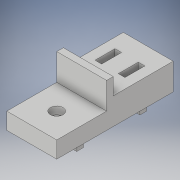
# Autodesk Inventor part: FixedFiber
Saved by Autodesk Inventor 2019 (Build 230136000, 136)
## iProperties
Created: 2019-06-10
Part Number: FixedFiber
Material: Generic
Document SubType Name: Modeling
Designer: aorfi
Density: 1 g/cm^3
Appearance: Default
Author: aorfi
Autodesk Inventor part; units mm, degrees
ref_plane "YZ Plane" through (0, 0, 0) normal (1, 0, 0) x (0, 1, 0)
ref_plane "XZ Plane" through (0, 0, 0) normal (0, 1, 0) x (-1, 0, 0)
ref_plane "XY Plane" through (0, 0, 0) normal (0, 0, 1) x (1, 0, 0)
sketch "Sketch1" plane through (0, 0, 0) normal (0, 1, 0) x (-1, 0, 0)
  line L0 (-7.5, 17.5) -> (7.5, 17.5)
  line L1 (7.5, 17.5) -> (7.5, -17.5)
  line L2 (7.5, -17.5) -> (-7.5, -17.5)
  line L3 (-7.5, -17.5) -> (-7.5, 17.5)
  line L4 (-7.5, 17.5) -> (7.5, -17.5) construction
  line L5 (7.5, 17.5) -> (-7.5, -17.5) construction
  point P0 (0, 0)
  dimension "d0" = 35
  dimension "d1" = 15
  constraints: 12 end point, 2 midpoint, 2 parallel, 1 horizontal, 1 perpendicular
  measures "d0" distance of L0.end L1.end
  measures "d1" distance of L1.end L2.end
extrude "Extrusion1" add sketch "Sketch1" along normal mid plane 8
sketch "Sketch4" plane through (0, 4, 0) normal (0, 1, 0) x (1, 0, 0)
  line L0 (-7.5, -2.5) -> (7.5, -2.5)
  line L1 (7.5, -2.5) -> (7.5, -0.5)
  line L2 (7.5, -0.5) -> (-7.5, -0.5)
  line L3 (-7.5, -0.5) -> (-7.5, -2.5)
  line L4 (-7.5, -17.5) -> (7.5, -17.5) projected
  line L5 (-7.5, 17.5) -> (-7.5, -17.5) projected
  line L6 (7.5, -17.5) -> (7.5, 17.5) projected
  dimension "d57" = 2
  dimension "d58" = 15
  constraints: 8 end point, 2 collinear, 2 parallel, 1 horizontal, 1 perpendicular
  measures "d57" distance of L2.end L0.start
  measures "d58" distance between parallel lines of L4 L0
extrude "Extrusion3" add sketch "Sketch4" along normal blind 5 contours L3 L2 L1 L0
sketch "Sketch5" plane through (0, 4, 0) normal (0, 1, 0) x (1, 0, 0)
  line L0 (-4.5, 12) -> (-2.5, 12)
  line L1 (-2.5, 12) -> (-2.5, 6)
  line L2 (-2.5, 6) -> (-4.5, 6)
  line L3 (-4.5, 6) -> (-4.5, 12)
  line L4 (4.5, 12) -> (2.5, 12)
  line L5 (2.5, 12) -> (2.5, 6)
  line L6 (2.5, 6) -> (4.5, 6)
  line L7 (4.5, 6) -> (4.5, 12)
  line L8 (-3.5, 9) -> (3.5, 9) construction
  line L9 (7.5, -0.5) -> (-7.5, -0.5) construction
  line L10 (-7.5, 12.8654) -> (-7.5, 4.5) construction
  line L11 (-7.5, 4.5) -> (-22.5, 4.5) construction
  line L12 (7.5, -0.5) -> (-7.5, -0.5) projected
  point P0 (0, -0.5)
  point P1 (0, 9)
  point P2 (3.5, 12)
  point P3 (-3.5, 12)
  point P4 (-2.5, 9)
  point P5 (0, 0)
  dimension "d20" = 6
  dimension "d21" = 2
  dimension "d22" = 5
  dimension "d26" = 1.5
  dimension "d31" = 7
  constraints: 24 end point, 5 midpoint, 4 parallel, 4 vertical alignment, 3 horizontal, 3 point on line, 2 collinear, 2 perpendicular
  measures "d20" distance of L2.end L0.start
  measures "d21" distance of L0.start L0.end
  measures "d22" distance between parallel lines of L9 L11
  measures "d26" distance between parallel lines of L2 L11
  measures "d31" distance of L8.start L8.end
extrude "Extrusion4" cut sketch "Sketch5" against normal blind 3
sketch "Sketch7" plane through (-7.5, -4, -17.5) normal (-1, 0, 0) x (0, 0, 1)
  line L0 (20, 8) -> (35, 8) projected
  line L1 (20, 8) -> (35, 8)
  line L2 (35, 8) -> (35, 5)
  line L3 (35, 5) -> (20, 5)
  line L4 (20, 5) -> (20, 8)
  line L5 (35, 8) -> (35, 0) projected
  point P0 (17.5, 4)
  dimension "d59" = 3
  constraints: 8 end point, 2 parallel, 1 collinear, 1 horizontal, 1 perpendicular
  measures "d59" distance between parallel lines of L0 L3
extrude "Extrusion6" cut sketch "Sketch7" against normal through all
sketch "Sketch8" plane through (0, 4, 0) normal (0, 1, 0) x (1, 0, 0)
  line L0 (-7.5, -0.5) -> (-7, -0.5)
  line L1 (-7, -0.5) -> (-7, 1.5)
  line L2 (-7, 1.5) -> (-7.5, 1.5)
  line L3 (-7.5, 1.5) -> (-7.5, -0.5)
  dimension "d60" = 2
  dimension "d61" = 0.5
  constraints: 8 end point, 2 parallel, 1 coincident, 1 horizontal, 1 perpendicular
  measures "d60" distance of L0.end L1.end
  measures "d61" distance of L1.end L2.end
extrude "Extrusion7" add sketch "Sketch8" along normal blind 1
sketch "Sketch11" plane through (0, -4, 0) normal (0, -1, 0) x (1, 0, 0)
  line L0 (-6.5, 10.5) -> (-4.5, 10.5)
  line L1 (-4.5, 10.5) -> (-4.5, 8.5)
  line L2 (-4.5, 8.5) -> (-6.5, 8.5)
  line L3 (-6.5, 8.5) -> (-6.5, 10.5)
  line L4 (6.5, 10.5) -> (4.5, 10.5)
  line L5 (4.5, 10.5) -> (4.5, 8.5)
  line L6 (4.5, 8.5) -> (6.5, 8.5)
  line L7 (6.5, 8.5) -> (6.5, 10.5)
  line L8 (-6.5, -8.5) -> (-4.5, -8.5)
  line L9 (-4.5, -8.5) -> (-4.5, -10.5)
  line L10 (-4.5, -10.5) -> (-6.5, -10.5)
  line L11 (-6.5, -10.5) -> (-6.5, -8.5)
  line L12 (6.5, -8.5) -> (4.5, -8.5)
  line L13 (4.5, -8.5) -> (4.5, -10.5)
  line L14 (4.5, -10.5) -> (6.5, -10.5)
  line L15 (6.5, -10.5) -> (6.5, -8.5)
  line L16 (-5.5, 9.5) -> (5.5, 9.5) construction
  line L17 (-5.5, 9.5) -> (-5.5, -9.5) construction
  line L18 (-7.5, 17.5) -> (-7.5, -17.5) projected
  line L19 (7.5, 17.5) -> (-7.5, 17.5) projected
  point P0 (0, 0)
  point P1 (-5.5, 10.5)
  point P2 (5.5, 10.5)
  point P3 (0, 9.5)
  point P4 (-6.5, 9.5)
  point P5 (-6.5, -9.5)
  point P6 (-5.5, 0)
  dimension "d62" = 2
  dimension "d63" = 2
  dimension "d64" = 2
  dimension "d65" = 2
  dimension "d68" = 2
  dimension "d69" = 8
  constraints: 36 end point, 8 parallel, 6 collinear, 6 midpoint, 5 horizontal, 4 perpendicular, 3 point on line, 3 vertical alignment, 2 horizontal alignment, 1 vertical
  measures "d62" distance of L0.start L0.end
  measures "d63" distance of L2.end L0.start
  measures "d64" distance of L4.start L4.end
  measures "d65" distance of L11.start L11.end
  measures "d68" distance between parallel lines of L18 L17
  measures "d69" distance between parallel lines of L19 L16
extrude "Extrusion9" add sketch "Sketch11" along normal blind 2
sketch "Sketch13" plane through (-7.5, 1, 17.5) normal (0, 1, 0) x (1, 0, 0)
  line L0 (15, 15) -> (15, 0) projected
  line L1 (15, 0) -> (0, 0) projected
  point P0 (7.5, 17.5)
  point P1 (7.5, 7.5)
  point P2 (15, 7.5)
  point P3 (7.5, 0)
  constraints: 2 midpoint, 1 horizontal alignment, 1 vertical alignment
hole "Hole3" at (0, 1, 10) direction (0, -1, 0) diameter 3.797 end through all clearance for "Flat Head Machine Screw (82)" size "#6" standard "Ansi Unified Screw Threads"
sketch "Sketch12" plane through (0, -4, 0) normal (0, -1, 0) x (1, 0, 0)
  line L0 (-3.937, 12.273) -> (0, 14.5461)
  line L1 (0, 14.5461) -> (3.937, 12.273)
  line L2 (3.937, 12.273) -> (3.937, 7.727)
  line L3 (3.937, 7.727) -> (0, 5.4539)
  line L4 (0, 5.4539) -> (-3.937, 7.727)
  line L5 (-3.937, 7.727) -> (-3.937, 12.273)
  line L6 (7.5, 17.5) -> (-7.5, 17.5) projected
  circle A0 centre (0, 10) radius 1.8985 projected
  point P0 (0, 0)
  point P1 (0, 10)
  dimension "d72" = 7.874
  constraints: 12 end point, 1 coincident, 1 vertical, 1 vertical alignment, 13 other
  measures "d72" distance between parallel lines of L2 L5
extrude "Extrusion10" cut sketch "Sketch12" against normal blind 2.7
equation "\"d63\" = d62"
equation "\"d64\" = d62"
equation "\"d65\" = d62"
body "Solid1"
